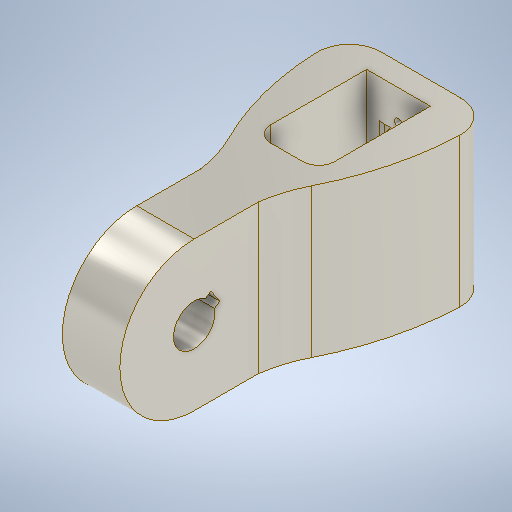
# Autodesk Inventor part: Link Three
Saved by Autodesk Inventor 2025.2 (Build 292293000, 293)
## iProperties
Created: 2025-03-05
Part Number: Link Three
Material: ABS Plastic
Document SubType Name: Modeling
Designer: abdal
Density: 1.06 g/cm^3
Appearance: Titanium
Mass: 137.373 g
Surface Area: 182.482 cm^2
Volume: 129.597 cm^3
Author: abdal
Autodesk Inventor part; units mm, degrees
ref_plane "YZ Plane" through (0, 0, 0) normal (1, 0, 0) x (0, 1, 0)
ref_plane "XZ Plane" through (0, 0, 0) normal (0, 1, 0) x (-1, 0, 0)
ref_plane "XY Plane" through (0, 0, 0) normal (0, 0, 1) x (1, 0, 0)
sketch "Sketch28" plane through (0, 0, 0) normal (1, 0, 0) x (0, 1, 0)
  circle A0 centre (0, 0) radius 6.5
  arc A1 (23.289, 0) -> (-23.289, 0) centre (0, 0) ccw
  line L0 (23.289, 0) -> (23.289, -80)
  line L1 (-23.289, 0) -> (-23.289, -80)
  line L2 (23.289, -80) -> (-23.289, -80)
  dimension "d103" = 13
  dimension "d104" = 46.578
  dimension "d105" = 80
  dimension "d106" = 80
  constraints: 6 end point, 2 centre point, 2 coincident, 2 point on circle, 2 tangent, 2 vertical
  measures "d103" diameter of A0
  measures "d104" diameter of A1
  measures "d105" distance of L0.start L0.end
  measures "d106" distance of L1.start L1.end
extrude "Extrusion23" add sketch "Sketch28" along normal blind 18
sketch "Sketch29" plane through (0, 23.289, 0) normal (0, 1, 0) x (1, 0, 0)
  line L0 (31.5, 80) -> (-13.5, 80)
  line L1 (-13.5, 80) -> (-13.5, 45)
  line L2 (-13.5, 45) -> (31.5, 45)
  line L3 (31.5, 45) -> (31.5, 80)
  line L4 (0, 80) -> (18, 80) projected
  line L5 (18, 0) -> (18, 80) projected
  arc A0 (31.5, 45) -> (18, 20) centre (57.6517, 14.7331) ccw
  line L6 (9, 88.5963) -> (9, -26.2001) construction
  arc A1 (0, 20) -> (-13.5, 45) centre (-39.6517, 14.7331) ccw
  line L7 (0, 80) -> (0, 0) projected
  point P0 (9, 80)
  point P1 (9, 45)
  point P2 (0, 45)
  point P3 (18, 45)
  dimension "d109" = 45
  dimension "d110" = 0
  dimension "d111" = 35
  dimension "d112" = 22.5
  dimension "d115" = 40
  dimension "d116" = 25
  constraints: 10 end point, 4 point on circle, 2 centre point, 2 midpoint, 2 parallel, 2 symmetric about line, 1 horizontal, 1 perpendicular, 1 point on line, 1 vertical, 1 other
  measures "d109" distance of L0.start L0.end
  measures "d110" distance between parallel lines of L4 L0
  measures "d111" distance of L2.end L0.start
  measures "d112" distance of point (9, 80) L0.start
  measures "d115" radius of A0
  measures "d116" distance from line of L2 A0.end
extrude "Extrusion24" add sketch "Sketch29" against normal up to surface (46.578 mm away)
fillet "Fillet9" radius 90 2 edges at (31.5, 0, -45) (-13.5, 0, -45)
sketch "Sketch30" plane through (0, 23.289, 0) normal (0, 1, 0) x (1, 0, 0)
  line L0 (19, 73) -> (-1, 73)
  line L1 (-1, 73) -> (-1, 38)
  line L2 (-1, 38) -> (19, 38)
  line L3 (19, 38) -> (19, 73)
  line L4 (-13.5, 80) -> (31.5, 80) projected
  point P0 (0, 0)
  dimension "d120" = 7
  dimension "d121" = 20
  dimension "d122" = 12.5
  dimension "d123" = 35
  constraints: 8 end point, 2 parallel, 1 horizontal, 1 perpendicular
  measures "d120" distance between parallel lines of L4 L0
  measures "d121" distance between parallel lines of L1 L3
  measures "d122" distance from line of L4.end L3
  measures "d123" distance between parallel lines of L0 L2
extrude "Extrusion25" cut sketch "Sketch30" against normal through all
fillet "Fillet10" radius 5 2 edges at (19, 0, -38) (-1, 0, -38)
fillet "Fillet11" radius 10 2 edges at (-13.5, 0, -80) (31.5, 0, -80)
sketch "Sketch31" plane through (21.4392, -23.289, -80) normal (0, 0, -1) x (-1, 0, 0)
  arc A0 (15.3892, 23.5545) -> (9.4892, 23.5545) centre (12.4392, 28.664) ccw projected
  line L0 (15.3892, 23.5545) -> (15.3892, 22.764) projected
  arc A1 (9.4892, 22.764) -> (15.3892, 22.764) centre (12.4392, 22.764) ccw projected
  line L1 (9.4892, 22.764) -> (9.4892, 23.5545) projected
  point P0 (21.4392, 23.289)
extrude "Extrusion26" cut sketch "Sketch31" against normal blind 20
sketch "Sketch34" plane through (-1, 23.289, -73) normal (0, 0, 1) x (1, 0, 0)
  line L0 (3.925, -12.014) -> (16.075, -12.014)
  line L1 (16.075, -12.014) -> (16.075, -34.564)
  line L2 (16.075, -34.564) -> (3.925, -34.564)
  line L3 (3.925, -34.564) -> (3.925, -12.014)
  line L4 (1, 0) -> (19, 0) projected
  arc A0 (12.95, -23.0235) -> (7.05, -23.0235) centre (10, -17.914) ccw projected
  point P0 (1, -23.289)
  point P1 (10, 0)
  dimension "d130" = 12.014
  dimension "d131" = 22.55
  dimension "d132" = 12.15
  dimension "d133" = 6.075
  constraints: 8 end point, 2 parallel, 1 horizontal, 1 midpoint, 1 perpendicular
  measures "d130" distance from line of point (10, 0) L0
  measures "d131" distance between parallel lines of L2 L0
  measures "d132" distance between parallel lines of L3 L1
  measures "d133" distance from line of A0.centre L3
extrude "Extrusion27" cut sketch "Sketch34" against normal blind 1.65
sketch "Sketch36" plane through (-1, 23.289, -73) normal (0, 0, 1) x (1, 0, 0)
  arc A0 (10.5833, -38.1445) -> (9.4167, -38.1445) centre (10, -37.039) ccw projected
  arc A1 (9.4167, -8.4335) -> (10.5833, -8.4335) centre (10, -9.539) ccw projected
  circle A2 centre (10, -9.539) radius 1.25
  circle A3 centre (10, -37.039) radius 1.25
  point P0 (1, -23.289)
  point P1 (10.5833, -8.4335)
  point P2 (9.4167, -8.4335)
  point P3 (9.4167, -38.1445)
  point P4 (10.5833, -38.1445)
  constraints: 2 centre point, 2 coincident, 2 concentric
extrude "Extrusion28" cut sketch "Sketch36" against normal through all
sketch "Sketch37" plane through (0, 0, 0) normal (-1, 0, 0) x (0, 0, 1)
  line L0 (-6.3739, 1.2741) -> (-8.0335, 2.3902) projected
  line L1 (-3.5835, 5.423) -> (-5.243, 6.5392) projected
  line L2 (-5.243, 6.5392) -> (-8.0335, 2.3902) projected
  circle A0 centre (0, 0) radius 6.5 projected
extrude "Extrusion29" cut sketch "Sketch37" against normal through all
sketch "Sketch38" plane through (0, 23.289, 0) normal (0, 1, 0) x (1, 0, 0)
  line L0 (-25.331, 0) -> (24.4324, 0)
  line L1 (0, 0) -> (18, 0) projected
  line L2 (9, 31.2847) -> (9, -25.5557)
  line L3 (0, -23.289) -> (18, -23.289) projected
  line L4 (14, 38) -> (4, 38) projected
  arc A0 (-1, 43) -> (4, 38) centre (4, 43) ccw projected
  line L5 (-1, 43) -> (-1, 73) projected
  line L6 (-1, 73) -> (19, 73) projected
  line L7 (19, 73) -> (19, 43) projected
  arc A1 (14, 38) -> (19, 43) centre (14, 43) ccw projected
  arc A2 (31.4316, 69.6103) -> (21.4392, 80) centre (21.4392, 70) ccw projected
  line L8 (-3.4392, 80) -> (21.4392, 80) projected
  arc A3 (-3.4392, 80) -> (-13.4316, 69.6103) centre (-3.4392, 70) ccw projected
  arc A4 (-13.4316, 69.6103) -> (-3.9127, 32.6976) centre (76.5, 73.1178) ccw projected
  arc A5 (0, 20) -> (-3.9127, 32.6976) centre (-39.6517, 14.7331) ccw projected
  line L9 (0, 20) -> (0, 0) projected
  line L10 (0, 0) -> (18, 0) projected
  line L11 (18, 20) -> (18, 0) projected
  arc A6 (21.9127, 32.6976) -> (18, 20) centre (57.6517, 14.7331) ccw projected
  arc A7 (21.9127, 32.6976) -> (31.4316, 69.6103) centre (-58.5, 73.1178) ccw projected
  circle A8 centre (9, 0) radius 2.5
  dimension "d140" = 0
  dimension "d141" = 9
  dimension "d142" = 5
  constraints: 4 end point, 1 centre point, 1 horizontal, 1 midpoint, 1 perpendicular
  measures "d140" distance between parallel lines of L1 L0
  measures "d141" distance between parallel lines of L9 L2
  measures "d142" diameter of A8
body "Solid2"
